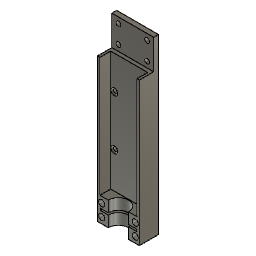
platform_bottom_10cc v2 (Autodesk Fusion 360 design; units mm, degrees)
Autodesk Fusion 360 part; units mm, degrees
sketch "スケッチ1" plane through (0, 0, 0) normal (0, 0, 1) x (1, 0, 0)
  line L0 (-17.5, 11) -> (17.5, 11)
  line L1 (17.5, 11) -> (17.5, 0)
  line L2 (17.5, 0) -> (-17.5, 0)
  line L3 (-17.5, 0) -> (-17.5, 11)
  dimension "d1" = 35
  dimension "d2" = 11
  constraint horizontal L0
  constraint vertical L1
  constraint horizontal L2
  constraint vertical L3
  constraint midpoint origin L2
  measures "d1" distance of L0.start L0.end
  measures "d2" distance of L0.start L2.end
extrude "押し出し1" add sketch "スケッチ1" along normal blind 120
sketch "スケッチ2" plane through (0, 0, 0) normal (0, 0, -1) x (1, 0, 0)
  line L0 (17.5, 0) -> (-17.5, 0)
  line L1 (-17.5, 0) -> (-17.5, -11)
  line L2 (-17.5, -11) -> (17.5, -11)
  line L3 (17.5, -11) -> (17.5, 0)
  circle A0 centre (0, 0) radius 8.5
  dimension "d5" = 17
  constraint coincident A0.centre origin
  measures "d5" diameter of A0
extrude "押し出し2" cut sketch "スケッチ2" against normal blind 20 contours L0 A0 picked at (-2.4352, -2.8535)
sketch "スケッチ3" plane through (0, 0, 120) normal (0, 0, 1) x (-1, 0, 0)
  line L0 (17.5, 0) -> (-17.5, 0)
  line L1 (-17.5, 0) -> (-17.5, -11)
  line L2 (-17.5, -11) -> (17.5, -11)
  line L3 (17.5, -11) -> (17.5, 0)
  line L4 (15.5, -9) -> (-15.5, -9)
  line L5 (-15.5, -9) -> (-15.5, 0)
  line L6 (-15.5, 0) -> (15.5, 0)
  line L7 (15.5, 0) -> (15.5, -9)
  dimension "d8" = 2
  dimension "d9" = 31
  constraint horizontal L4
  constraint vertical L5
  constraint horizontal L6
  constraint vertical L7
  constraint coincident L0 L5.end
  constraint midpoint origin L6
  measures "d8" distance of L2 L4
  measures "d9" distance of L5 L7
extrude "押し出し3" cut sketch "スケッチ3" against normal blind 100 contours L0 L4 L5 L6 L7
ref_plane "作業平面1" through (0, 5.5, 9) normal (0, 0, -1) x (-1, 0, 0)
sketch "スケッチ5" plane through (0, 11, 0) normal (0, 1, 0) x (-1, 0, 0)
  line L0 (-17.5, 0) -> (17.5, 0)
  line L1 (17.5, 0) -> (17.5, 120)
  line L2 (17.5, 120) -> (-17.5, 120)
  line L3 (-17.5, 120) -> (-17.5, 0)
  line L4 (-17.5, 130) -> (17.5, 130)
  line L5 (17.5, 130) -> (17.5, 120)
  line L6 (17.5, 120) -> (-17.5, 120)
  line L7 (-17.5, 120) -> (-17.5, 130)
  line L8 (-17.5, 125) -> (17.5, 125) construction
  circle A0 centre (12, 125) radius 2
  circle A1 centre (-12, 125) radius 2
  dimension "d16" = 4
  dimension "d17" = 4
  dimension "d18" = 24
  dimension "d19" = 10
  dimension "d20" = 5.5
  constraint horizontal L4
  constraint vertical L5
  constraint horizontal L6
  constraint vertical L7
  constraint collinear L2 L6
  constraint midpoint L7 L8.start
  constraint midpoint L5 L8.end
  constraint coincident L8 A0.centre
  constraint coincident L8 A1.centre
  constraint collinear L3 L7
  constraint collinear L1 L5
  measures "d16" diameter of A1
  measures "d17" diameter of A0
  measures "d18" distance of A0.centre A1.centre
  measures "d19" distance of L4.start L2.end
  measures "d20" distance of L8.end A0.centre
extrude "押し出し5" add sketch "スケッチ5" against normal blind 2 contours L2 L4 L5 L6 L7
sketch "スケッチ8" plane through (0, 0, 0) normal (0, -1, 0) x (1, 0, 0)
  line L0 (-8.5, 20) -> (-15.5, 20)
  line L1 (-15.5, 20) -> (-15.5, 120)
  line L2 (-15.5, 120) -> (-17.5, 120)
  line L3 (-17.5, 120) -> (-17.5, 0)
  line L4 (-17.5, 0) -> (-8.5, 0)
  line L5 (-8.5, 0) -> (-8.5, 20)
  circle A0 centre (-14, 15) radius 2.55
  line L6 (18.5, 15) -> (-17.5, 15) construction
  line L7 (17.541, 5) -> (-17.5, 5) construction
  line L8 (15.5, 20) -> (8.5, 20) construction
  circle A1 centre (14, 15) radius 2.55
  circle A2 centre (14, 5) radius 2.55
  circle A3 centre (-14, 5) radius 2.55
  line L9 (17.5, 0) -> (17.5, 120)
  dimension "d30" = 5
  dimension "d31" = 10
  dimension "d32" = 5.1
  dimension "d33" = 5.1
  dimension "d34" = 5.1
  dimension "d35" = 5.1
  dimension "d36" = 3.5
  dimension "d37" = 3.5
  dimension "d38" = 3.5
  dimension "d39" = 3.5
  constraint coincident L3 L6.end
  constraint perpendicular L3 L6
  constraint coincident L3 L7.end
  constraint perpendicular L3 L7
  constraint coincident L6 A1.centre
  constraint coincident L7 A2.centre
  constraint coincident L7 A3.centre
  constraint coincident A0.centre L6
  measures "d30" distance of L6 L8
  measures "d31" distance of L6 L7
  measures "d32" diameter of A0
  measures "d33" diameter of A1
  measures "d34" diameter of A2
  measures "d35" diameter of A3
  measures "d36" distance of A0.centre L6.end
  measures "d37" distance of L3 A3.centre
  measures "d38" distance of A1.centre L9
  measures "d39" distance of A2.centre L9
extrude "押し出し8" cut sketch "スケッチ8" against normal blind 15 contours A0 | A1 | A2 | A3
move_face "OffsetFaces1" offset 3 1 faces at (-3.8517, 11, 52.6741)
sketch "Sketch9" plane through (0, 9, 0) normal (0, -1, 0) x (1, 0, 0)
  circle A0 centre (12, 125) radius 2
  circle A1 centre (-12, 125) radius 2
  line L0 (-15.5, 120) -> (-15.5, 20)
  line L1 (-15.5, 20) -> (15.5, 20)
  line L2 (15.5, 20) -> (15.5, 120)
  line L3 (15.5, 120) -> (17.5, 120)
  line L4 (17.5, 120) -> (17.5, 130)
  line L5 (17.5, 130) -> (-17.5, 130)
  line L6 (-17.5, 130) -> (-17.5, 120)
  line L7 (-17.5, 120) -> (-15.5, 120)
  point P0 (12.5, 50)
  point P1 (-12.5, 50)
  point P2 (-12.5, 92)
  point P3 (12.5, 92)
  constraint horizontal P0 P1
  constraint vertical P1 P2
hole "Hole1" at (-12.5, 9, 92) at (12.5, 9, 92) at (12.5, 9, 50) at (-12.5, 9, 50) direction (0, 1, 0) diameter 3.4 depth 9 tip angle 118 countersink diameter 5.6 countersink angle 90
ref_plane "WorkPlane2" through (0, 0, 10) normal (0, 0, 1) x (1, 0, 0)
sketch "Sketch10" plane through (0, 0, 10) normal (0, 0, 1) x (1, 0, 0)
  line L0 (0, 0) -> (15.25, 0)
  line L1 (15.25, 0) -> (15.25, 8)
  line L2 (15.25, 8) -> (0, 10)
  line L3 (0, 0) -> (-15.25, 0)
  line L4 (-15.25, 0) -> (-15.25, 8)
  line L5 (-15.25, 8) -> (0, 10)
  dimension "d60" = 15.25
  dimension "d61" = 8
  constraint coincident L0.start L3.start
  constraint horizontal L0
  constraint vertical L1
  measures "d60" distance of L0.start L0.end
  measures "d61" distance of L0.end L1.end
extrude "Extrude9" cut sketch "Sketch10" along normal blind 0.85 and the other way blind 0.85
sketch "Sketch11" plane through (0, 9, 0) normal (0, -1, 0) x (1, 0, 0)
  circle A0 centre (12.5, 50) radius 2.8
  circle A1 centre (-12.5, 92) radius 2.8
  circle A2 centre (12.5, 92) radius 2.8
  circle A3 centre (-12.5, 50) radius 2.8
  circle A4 centre (-12, 125) radius 2
  circle A5 centre (12, 125) radius 2
  line L0 (-15.5, 120) -> (-15.5, 20)
  line L1 (-15.5, 20) -> (15.5, 20)
  line L2 (15.5, 20) -> (15.5, 120)
  line L3 (15.5, 120) -> (17.5, 120)
  line L4 (17.5, 120) -> (17.5, 130)
  line L5 (17.5, 130) -> (-17.5, 130)
  line L6 (-17.5, 130) -> (-17.5, 120)
  line L7 (-17.5, 120) -> (-15.5, 120)
  line L8 (-17.5, 130) -> (17.5, 130)
  line L9 (17.5, 130) -> (17.5, 120)
  line L10 (17.5, 120) -> (-17.5, 120)
  line L11 (-17.5, 120) -> (-17.5, 130)
  constraint horizontal L8
  constraint vertical L9
  constraint horizontal L10
  constraint vertical L11
  constraint coincident L3.end L4.start
  constraint coincident L5.end L6.start
extrude "Extrude10" cut sketch "Sketch11" against normal blind 3 contours L3 L4 L5 L6 L7 L8 L9 L10 L11
move_face "OffsetFaces2" offset 2 1 faces at (-3.9094, 14, 64.5049)
move_face "OffsetFaces3" offset 15 1 faces at (5.8333, 13.3333, 130)
sketch "Sketch12" plane through (0, 12, 0) normal (0, -1, 0) x (1, 0, 0)
  circle A0 centre (12, 125) radius 2
  circle A1 centre (-12, 125) radius 2
  line L0 (-17.5, 120) -> (17.5, 120)
  line L1 (17.5, 120) -> (17.5, 145)
  line L2 (17.5, 145) -> (-17.5, 145)
  line L3 (-17.5, 145) -> (-17.5, 120)
  point P0 (-12, 140)
  point P1 (12, 140)
  constraint horizontal P0 P1
hole "Hole2" at (-12, 12, 140) at (12, 12, 140) direction (0, 1, 0) diameter 4 depth 5 tip angle 118
